skadis_bracket_right (Autodesk Fusion 360 design; units mm, degrees)
part number: 2026-09-05-18-11-34-603
Autodesk Fusion 360 part; units mm, degrees
sketch "Plate" plane through (0, 0, 0) normal (0, 1, 0) x (1, 0, 0)
  line L0 (0, 0) -> (5.4, 0)
  line L1 (5.4, 0) -> (5.4, -60)
  line L2 (5.4, -60) -> (0, -60)
  line L3 (0, -60) -> (0, 0)
  dimension "d242" = 5.4
  dimension "d243" = 60
  constraint coincident L0.start L3.end
  constraint horizontal L0
  constraint horizontal L2
  constraint vertical L1
  constraint vertical L3
  measures "d242" horizontal distance of L0.start L1.end
  measures "d243" vertical distance of L0.start L1.end
extrude "Plate (1)" add sketch "Plate" along normal mid plane 28 from surface at -2
sketch "Hook profile" plane through (0, 0, 0) normal (0, 1, 0) x (1, 0, 0)
  line L0 (0, -58) -> (-8.3, -58)
  line L1 (-8.3, -58) -> (-8.3, -41)
  line L2 (-8.3, -41) -> (-5.3, -41)
  line L3 (-5.3, -41) -> (-3.8, -42.5)
  line L4 (-3.8, -42.5) -> (-3.8, -53)
  line L5 (-3.8, -53) -> (0, -53)
  line L6 (0, -53) -> (0, -58)
  dimension "d247" = 58
  dimension "d248" = 8.3
  dimension "d249" = 3.8
  dimension "d250" = 5
  dimension "d251" = 10.5
  dimension "d252" = 1.5
  dimension "d253" = 1.5
  constraint horizontal L0
  constraint horizontal L2
  constraint horizontal L5
  constraint vertical L1
  constraint vertical L4
  constraint vertical L6
  constraint coincident origin L6
  measures "d247" vertical distance of origin L0.start
  measures "d248" horizontal distance of L0.start L0.end
  measures "d249" horizontal distance of L4.end L5.end
  measures "d250" vertical distance of L0.start L5.end
  measures "d251" vertical distance of L3.end L4.end
  measures "d252" horizontal distance of L2.end L3.end
  measures "d253" vertical distance of L2.end L3.end
extrude "Hook profile (1)" add sketch "Hook profile" along normal mid plane 2.4
pattern_linear "Hook rows" count 2 spacing 25.4 along (0, 0, -1) count 3 spacing 0 along (0, 0, 1) of "Hook profile (1)"
sketch "Peg profile" plane through (0, 0, 0) normal (0, 1, 0) x (1, 0, 0)
  line L0 (5.4, -45) -> (12.2, -45)
  line L1 (12.2, -45) -> (12.2, -55.4)
  line L2 (12.2, -55.4) -> (11.6, -56)
  line L3 (11.6, -56) -> (10.2, -56)
  line L4 (10.2, -56) -> (10.2, -49)
  line L5 (10.2, -49) -> (5.4, -49)
  line L6 (5.4, -49) -> (5.4, -45)
  dimension "d260" = 5.4
  dimension "d261" = 45
  dimension "d262" = 12.2
  dimension "d263" = 55.4
  dimension "d264" = 11.6
  dimension "d265" = 56
  dimension "d266" = 10.2
  dimension "d267" = 49
  constraint horizontal L0
  constraint horizontal L3
  constraint horizontal L5
  constraint vertical L1
  constraint vertical L4
  constraint vertical L6
  measures "d260" horizontal distance of origin L0.start
  measures "d261" vertical distance of origin L0.start
  measures "d262" horizontal distance of origin L0.end
  measures "d263" vertical distance of origin L1.end
  measures "d264" horizontal distance of origin L2.end
  measures "d265" vertical distance of origin L2.end
  measures "d266" horizontal distance of origin L3.end
  measures "d267" vertical distance of origin L4.end
extrude "Peg profile (1)" add sketch "Peg profile" along normal mid plane 4.7 from surface at -7.52
pattern_linear "Peg rows" count 2 spacing 40 along (0, 0, -1) count 3 spacing 0 along (0, 0, 1) of "Peg profile (1)"
fillet "Peg bearing fillets" radius 1.5 4 edges at (7.8, -9.87, 9) (7.8, -5.17, 9) (7.8, -9.87, 49) (7.8, -5.17, 49)
fillet "Prong front fillets" radius 1 4 edges at (12.2, -5.17, 50.2) (12.2, -5.17, 10.2) (12.2, -9.87, 10.2) (12.2, -9.87, 50.2)
equation "bracketWidth = 24.0 mm" comment "bracket width across the upright"
equation "plateThickness = 5.4 mm" comment "board rear face sits on this"
equation "plateHeight = 60.0 mm" comment "plate height"
equation "slotWidth = 3.2 mm" comment "measured upright slot width"
equation "slotPitchVertical = 25.4 mm" comment "1 inch, measured"
equation "faceMetalThickness = 2.0 mm" comment "upright face metal"
equation "hookTabWidth = slotWidth - 0.8 mm" comment "blade width through the slot"
equation "hookThroat = faceMetalThickness + 1.8 mm" comment "gap behind the plate"
equation "hookNeckHeight = 5.0 mm" comment "bears on the slot bottom edge"
equation "hookLipThickness = 4.5 mm" comment "lip behind the upright face"
equation "hookLipDrop = 12.0 mm" comment "engagement below the neck"
equation "hookLipChamfer = 1.5 mm" comment "lead-in past slot burrs"
equation "topHookNeckTop = 58.0 mm" comment "top hook row"
equation "hookRows = 2" comment "hook rows (pattern count)"
equation "boardThickness = 4.6 mm" comment "SKADIS panel thickness"
equation "boardSlotWidth = 5.0 mm" comment "SKADIS slot width"
equation "boardSlotHeight = 15.0 mm" comment "SKADIS slot height"
equation "boardPitch = 40.0 mm" comment "SKADIS grid pitch"
equation "pegWidth = boardSlotWidth - pegClearance" comment "peg width in the slot"
equation "pegRootLength = boardThickness + pegRootProud" comment "root through the board"
equation "pegRootHeight = 4.0 mm" comment "slot top edge bears on this"
equation "pegProngThickness = 2.0 mm" comment "prong in front of board"
equation "pegTotalHeight = boardSlotHeight - 4 mm" comment "prong rise above the root, and the lift needed to release"
equation "pegProngChamfer = 0.6 mm" comment "lead-in on the prong top"
equation "pegBearingFillet = 1.5 mm" comment "round on the root top edges the board bears on"
equation "topPegRootZ = 45.0 mm" comment "top peg root, above the plate foot"
equation "pegRows = 2" comment "pegs per bracket (pattern count)"
equation "pegOffsetY = -7.52 mm" comment "offset onto the board's 40 mm grid"
equation "plateInboardExtension = 4.0 mm" comment "extra plate toward the desk centre, where the peg crowds"
equation "pegClearance = 0.3 mm" comment "sliding fit across the slot"
equation "pegRootProud = 0.2 mm" comment "root past the board's front face"
equation "pegProngFrontFillet = 1.0 mm" comment "round on the prong's front corners, where fingers meet it"
equation "d242 = plateThickness"
equation "d243 = plateHeight"
equation "d244 = -plateInboardExtension / 2"
equation "d245 = bracketWidth + plateInboardExtension"
equation "d247 = topHookNeckTop"
equation "d248 = hookThroat + hookLipThickness"
equation "d249 = hookThroat"
equation "d250 = hookNeckHeight"
equation "d251 = hookLipDrop - hookLipChamfer"
equation "d252 = hookLipChamfer"
equation "d253 = hookLipChamfer"
equation "d254 = hookTabWidth"
equation "d256 = hookRows"
equation "d258 = -slotPitchVertical"
equation "d260 = plateThickness"
equation "d261 = topPegRootZ"
equation "d262 = plateThickness + pegRootLength + pegProngThickness"
equation "d263 = topPegRootZ + pegTotalHeight - pegProngChamfer"
equation "d264 = plateThickness + pegRootLength + pegProngThickness - pegProngChamfer"
equation "d265 = topPegRootZ + pegTotalHeight"
equation "d266 = plateThickness + pegRootLength"
equation "d267 = topPegRootZ + pegRootHeight"
equation "d268 = pegOffsetY"
equation "d269 = pegWidth"
equation "d271 = pegRows"
equation "d273 = -boardPitch"
equation "d276 = pegBearingFillet"
equation "d278 = pegProngFrontFillet"
named bodies: "skadis_bracket_right"
